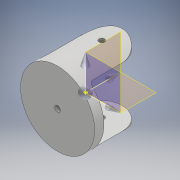
# Autodesk Inventor part: hlava
Saved by Autodesk Inventor 2017 (Build 210142000, 142)
## iProperties
Created: 2019-02-01
Part Number: hlava
Material: Generic
Document SubType Name: Modeling
Designer: Denis Kurka
Density: 1 g/cm^3
Appearance: Default
Author: Denis Kurka
Autodesk Inventor part; units mm, degrees
ref_plane "YZ Plane" through (0, 0, 0) normal (1, 0, 0) x (0, 1, 0)
ref_plane "XZ Plane" through (0, 0, 0) normal (0, 1, 0) x (-1, 0, 0)
ref_plane "XY Plane" through (0, 0, 0) normal (0, 0, 1) x (1, 0, 0)
sketch "Sketch1" plane through (0, 0, 0) normal (0, 1, 0) x (-1, 0, 0)
  circle A0 centre (0, 0) radius 20
  dimension "d0" = 40
  constraints: 1 centre point, 1 coincident
  measures "d0" diameter of A0
extrude "Extrusion1" add sketch "Sketch1" along normal blind 5
sketch "Sketch2" plane through (0, 5, 0) normal (0, 1, 0) x (1, 0, 0)
  circle A0 centre (0, 0) radius 20 projected
  line L0 (-12, 16) -> (12, 16)
  line L1 (-12, -16) -> (12, -16)
  dimension "d3" = 4
  dimension "d4" = 4
  constraints: 4 end point, 4 point on circle, 1 horizontal
  measures "d3" distance edge to line of A0 L0
  measures "d4" distance edge to line of A0 L1
extrude "Extrusion2" add sketch "Sketch2" along normal blind 30 contours L0 A0 | A0 L1
sketch "Sketch4" plane through (12, 5, 16) normal (0, 0, -1) x (-1, 0, 0)
  line L0 (24, 30) -> (24, 17.9)
  line L1 (0, 30) -> (0, 17.9)
  arc A0 (11.8923, 29.9) -> (0, 17.9) centre (12, 17.9005) ccw
  arc A1 (24, 17.9) -> (11.8923, 29.9) centre (12, 17.9005) ccw
  line L2 (0, 30) -> (24, 30)
  point P0 (12, -5)
  dimension "d10" = 12.1
  dimension "d11" = 12.1
  dimension "d12" = 12
  dimension "d13" = 12
  constraints: 6 end point, 4 point on circle, 2 centre point, 1 horizontal, 1 vertical
  measures "d10" distance of L0.start L0.end
  measures "d11" distance of L1.start L1.end
  measures "d12" radius of A0
  measures "d13" radius of A1
extrude "Extrusion3" cut sketch "Sketch4" against normal blind 25
sketch "Sketch5" plane through (-12, 5, -16) normal (0, 0, 1) x (1, 0, 0)
  line L0 (24, 30) -> (24, 17.9)
  line L1 (0, 30) -> (0, 17.9)
  arc A0 (12, 29.9) -> (0, 17.9) centre (12, 17.9) ccw
  arc A1 (24, 17.9) -> (12, 29.9) centre (12, 17.9) ccw
  line L2 (24, 30) -> (0, 30) projected
  line L3 (0, 30) -> (24, 30)
  point P0 (12, -5)
  dimension "d16" = 12.1
  dimension "d17" = 12.1
  dimension "d18" = 12
  dimension "d19" = 12
  constraints: 6 end point, 4 point on circle, 2 centre point, 1 horizontal, 1 vertical
  measures "d16" distance of L0.start L0.end
  measures "d17" distance of L1.start L1.end
  measures "d18" radius of A0
  measures "d19" radius of A1
extrude "Extrusion4" cut sketch "Sketch5" against normal blind 25
sketch "Sketch6" plane through (-12, 5, -16) normal (0, 0, 1) x (1, 0, 0)
  circle A0 centre (12, 18.8433) radius 1.5
  line L0 (0, 0) -> (0, 18.8433)
  line L1 (0, 18.8433) -> (23.891, 18.8433)
  point P0 (12, -5)
  dimension "d22" = 3
  dimension "d23" = 12
  dimension "d24" = 0
  constraints: 4 end point, 1 centre point, 1 horizontal, 1 vertical
  measures "d22" diameter of A0
  measures "d23" distance from line of L0 A0.centre
  measures "d24" distance from line of L1 A0.centre
extrude "Extrusion5" cut sketch "Sketch6" along normal mid plane 500
fillet "Fillet1" radius 2 2 edges at (0, 5, 16) (0, 5, -16)
sketch "Sketch7" plane through (0, 5, 0) normal (0, 1, 0) x (1, 0, 0)
  circle A0 centre (0, 0) radius 1.5
  dimension "d28" = 3
  constraints: 1 centre point, 1 coincident
  measures "d28" diameter of A0
extrude "Extrusion6" cut sketch "Sketch7" against normal blind 10
body "Solid1"
